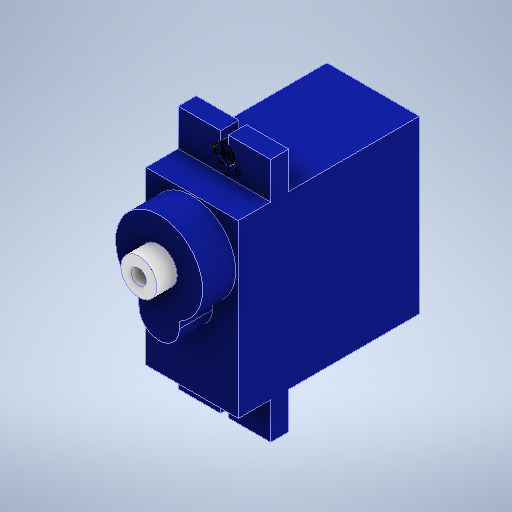
# Autodesk Inventor part: SG90 Servo
Saved by Autodesk Inventor 2025.1 (Build 291241000, 241)
## iProperties
Created: 2024-10-27
Part Number: SG90 Servo
Material: Generic
Document SubType Name: Modeling
Designer: jerem
Density: 1 g/cm^3
Appearance: Default
Author: jerem
Autodesk Inventor part; units mm, degrees
ref_plane "YZ Plane" through (0, 0, 0) normal (1, 0, 0) x (0, 1, 0)
ref_plane "XZ Plane" through (0, 0, 0) normal (0, 1, 0) x (-1, 0, 0)
ref_plane "XY Plane" through (0, 0, 0) normal (0, 0, 1) x (1, 0, 0)
sketch "Sketch1" plane through (0, 0, 0) normal (0, 0, 1) x (1, 0, 0)
  line L0 (6.15, -11.4) -> (-6.15, -11.4)
  line L1 (-6.15, -11.4) -> (-6.15, 11.4)
  line L2 (-6.15, 11.4) -> (6.15, 11.4)
  line L3 (6.15, 11.4) -> (6.15, -11.4)
  line L4 (6.15, -11.4) -> (-6.15, 11.4) construction
  line L5 (-6.15, -11.4) -> (6.15, 11.4) construction
  line L6 (-6.15, 11.4) -> (-6.15, 16.3)
  line L7 (6.15, 16.3) -> (6.15, 11.4)
  line L8 (-6.15, -11.4) -> (-6.15, -16.3)
  line L9 (6.15, -16.3) -> (6.15, -11.4)
  arc A0 (-0.5, 15.1) -> (0.5, 15.1) centre (0, 13.9) ccw
  line L10 (0, 13.9) -> (0, 11.4) construction
  line L11 (-0.5, 16.3) -> (-0.5, 15.1)
  line L12 (0.5, 15.1) -> (0.5, 16.3)
  line L13 (-0.5, 15.1) -> (0.5, 15.1) construction
  line L14 (0, 13.9) -> (0, 15.1) construction
  line L15 (-6.15, 16.3) -> (-0.5, 16.3)
  line L16 (0.5, 16.3) -> (6.15, 16.3)
  arc A1 (0.5, -15.1) -> (-0.5, -15.1) centre (0, -13.9) ccw
  line L17 (-0.5, -15.1) -> (-0.5, -16.3)
  line L18 (0.5, -15.1) -> (0.5, -16.3)
  line L19 (-0.5, -15.1) -> (0.5, -15.1) construction
  line L20 (0, -15.1) -> (0, -13.9) construction
  line L21 (0, -13.9) -> (0, -11.4) construction
  line L22 (-6.15, -16.3) -> (-0.5, -16.3)
  line L23 (0.5, -16.3) -> (6.15, -16.3)
  line L24 (0, 11.4) -> (0, 5.4) construction
  circle A2 centre (0, 5.4) radius 1
  circle A3 centre (0, 5.4) radius 2.4
  arc A4 (-2.7, -0.6) -> (2.7, -0.6) centre (0, -0.6) ccw
  line L25 (0, 5.4) -> (0, -0.6) construction
  line L26 (-2.7, -0.6) -> (-2.7, 0.2668)
  line L27 (2.7, -0.6) -> (2.7, 0.2668)
  arc A5 (2.7, 0.2668) -> (-2.7, 0.2668) centre (0, 5.4) ccw
  point P0 (0, 0)
  dimension "d0" = 22.8
  dimension "d1" = 12.3
  dimension "d4" = 2.6
  dimension "d5" = 2.5
  dimension "d6" = 1
  dimension "d7" = 4.9
  dimension "d8" = 2.5
  dimension "d9" = 1
  dimension "d10" = 2.6
  dimension "d11" = 4.9
  dimension "d14" = 6
  dimension "d15" = 2
  dimension "d16" = 4.8
  dimension "d17" = 5.4
  dimension "d18" = 6
  dimension "d19" = 5.8
  constraints: 57 end point, 15 perpendicular, 10 vertical, 8 point on circle, 6 centre point, 6 midpoint, 3 horizontal, 3 parallel, 2 coincident, 2 collinear, 2 tangent
  measures "d0" distance of L0.end L1.end
  measures "d1" distance of L1.end L2.end
  measures "d4" diameter of A0
  measures "d5" distance of L10.start L10.end
  measures "d6" distance between parallel lines of L12 L11
  measures "d7" distance between parallel lines of L2 L16
  measures "d8" distance of L20.end L21.end
  measures "d9" distance between parallel lines of L18 L17
  measures "d10" diameter of A1
  measures "d11" distance between parallel lines of L0 L23
  measures "d14" distance of L10.end L24.end
  measures "d15" diameter of A2
  measures "d16" diameter of A3
  measures "d17" diameter of A4
  measures "d18" distance of L25.start L25.end
  measures "d19" radius of A5
extrude "Extrusion1" add sketch "Sketch1" against normal blind 17.4 contours L0 L1 L2 L3 | A2 | A3 | L26 A5 L27 A4
extrude "Extrusion2" add sketch "Sketch1" along normal blind 2.4 contours L9 L23 L18 A1 L17 L22 L8 L0 | L0 L1 L2 L3 | L2 L6 L15 L11 A0 L12 L16 L7 | A2 | A3 | L26 A5 L27 A4
extrude "Extrusion3" add sketch "Sketch1" along normal blind 4.3 from surface at 2.4 contours L0 L1 L2 L3 | A2 | A3 | L26 A5 L27 A4
extrude "Extrusion4" add sketch "Sketch1" along normal blind 4.4 from surface at 6.7 contours A2 | A3 | L26 A5 L27 A4
extrude "Extrusion5" add sketch "Sketch1" along normal blind 2.7 from surface at 11.1 contours A3
sketch "Sketch2" plane through (0, 5.4, 11.1) normal (0, 0, 1) x (1, 0, 0)
  arc A0 (2.7, -5.1332) -> (-2.7, -5.1332) centre (0, 0) ccw projected
  line L0 (2.7, -5.1332) -> (2.7, -6) projected
  line L1 (-2.7, -6) -> (-2.7, -5.1332) projected
  arc A1 (-2.7, -6) -> (2.7, -6) centre (0, -6) ccw projected
  line L2 (6.15, -16.8) -> (-6.15, -16.8) projected
  line L3 (-6.15, -16.8) -> (6.15, -16.8) projected
  line L4 (6.15, -16.8) -> (-6.15, -16.8) projected
  line L5 (6.15, 6) -> (6.15, -16.8) projected
  line L6 (-6.15, 6) -> (6.15, 6) projected
  line L7 (-6.15, -16.8) -> (-6.15, 6) projected
  arc A2 (-2.7, -6) -> (2.7, -6) centre (0, -6) ccw projected
  line L8 (-2.7, -6) -> (-2.7, -5.1332) projected
  arc A3 (2.7, -5.1332) -> (-2.7, -5.1332) centre (0, 0) ccw projected
  line L9 (2.7, -5.1332) -> (2.7, -6) projected
  line L10 (-6.15, -16.8) -> (-6.15, 6) projected
  line L11 (6.15, -16.8) -> (-6.15, -16.8) projected
  line L12 (6.15, 6) -> (6.15, -16.8) projected
  line L13 (-6.15, 6) -> (6.15, 6) projected
  line L14 (-6.15, -16.8) -> (-6.15, 6) projected
  line L15 (-6.15, -16.8) -> (-6.15, -21.7) projected
  line L16 (-6.15, -16.8) -> (-6.15, -21.7) projected
  line L17 (-6.15, -16.8) -> (-6.15, 6) projected
  line L18 (-6.15, 10.9) -> (-6.15, 6) projected
  line L19 (-6.15, 10.9) -> (-6.15, 6) projected
  line L20 (6.15, 6) -> (6.15, -16.8) projected
  line L21 (6.15, -21.7) -> (6.15, -16.8) projected
  line L22 (6.15, -21.7) -> (6.15, -16.8) projected
  line L23 (6.15, 6) -> (6.15, -16.8) projected
  line L24 (6.15, 6) -> (6.15, 10.9) projected
  line L25 (6.15, 6) -> (6.15, 10.9) projected
  line L26 (6.15, -16.8) -> (-6.15, -16.8) projected
  line L27 (-6.15, -16.8) -> (-6.15, 6) projected
  line L28 (-6.15, 6) -> (6.15, 6) projected
  line L29 (6.15, 6) -> (6.15, -16.8) projected
  line L30 (-6.15, -16.8) -> (-6.15, 6) projected
  line L31 (6.15, 6) -> (6.15, -16.8) projected
  line L32 (-6.15, 6) -> (6.15, 6) projected
  line L33 (-6.15, -16.8) -> (6.15, -16.8) projected
  line L34 (6.15, -16.8) -> (-6.15, -16.8) projected
  line L35 (6.15, -16.8) -> (-6.15, -16.8) projected
  line L36 (6.15, -16.8) -> (-6.15, -16.8) projected
  line L37 (6.15, -21.7) -> (6.15, -16.8) projected
  line L38 (6.15, -21.7) -> (6.15, -16.8) projected
  line L39 (0.5, -20.5) -> (0.5, -21.7) projected
  line L40 (0.5, -20.5) -> (0.5, -21.7) projected
  line L41 (0.5, -20.5) -> (0.5, -21.7) projected
  line L42 (0.5, -21.7) -> (6.15, -21.7) projected
  line L43 (0.5, -21.7) -> (6.15, -21.7) projected
  line L44 (-6.15, -16.8) -> (-6.15, -21.7) projected
  line L45 (6.15, -16.8) -> (-6.15, -16.8) projected
  line L46 (-6.15, -16.8) -> (-6.15, -21.7) projected
  line L47 (-6.15, -21.7) -> (-0.5, -21.7) projected
  line L48 (-0.5, -21.7) -> (-0.5, -20.5) projected
  arc A4 (0.5, -20.5) -> (-0.5, -20.5) centre (0, -19.3) ccw projected
  line L49 (0.5, -20.5) -> (0.5, -21.7) projected
  line L50 (0.5, -21.7) -> (6.15, -21.7) projected
  line L51 (6.15, -21.7) -> (6.15, -16.8) projected
  line L52 (-6.15, -16.8) -> (6.15, -16.8) projected
  line L53 (6.15, -21.7) -> (6.15, -16.8) projected
  line L54 (0.5, -21.7) -> (6.15, -21.7) projected
  line L55 (0.5, -20.5) -> (0.5, -21.7) projected
  arc A5 (0.5, -20.5) -> (-0.5, -20.5) centre (0, -19.3) ccw projected
  line L56 (-0.5, -21.7) -> (-0.5, -20.5) projected
  line L57 (-6.15, -21.7) -> (-0.5, -21.7) projected
  line L58 (-6.15, -16.8) -> (-6.15, -21.7) projected
  line L59 (-6.15, -16.8) -> (-6.15, -21.7) projected
  line L60 (6.15, -16.8) -> (-6.15, -16.8) projected
  line L61 (-6.15, -21.7) -> (-0.5, -21.7) projected
  line L62 (-6.15, -21.7) -> (-0.5, -21.7) projected
  line L63 (-6.15, -21.7) -> (-0.5, -21.7) projected
  line L64 (0.5, -21.7) -> (6.15, -21.7) projected
  line L65 (-6.15, -21.7) -> (-0.5, -21.7) projected
  line L66 (-0.5, -21.7) -> (-0.5, -20.5) projected
  line L67 (-0.5, -21.7) -> (-0.5, -20.5) projected
  line L68 (-0.5, -21.7) -> (-0.5, -20.5) projected
  line L69 (-0.5, -21.7) -> (-0.5, -20.5) projected
  line L70 (0.5, -21.7) -> (6.15, -21.7) projected
  line L71 (-6.15, 10.9) -> (-6.15, 6) projected
  line L72 (-6.15, 10.9) -> (-6.15, 6) projected
  line L73 (6.15, 6) -> (6.15, 10.9) projected
  line L74 (6.15, 10.9) -> (0.5, 10.9) projected
  line L75 (0.5, 10.9) -> (0.5, 9.7) projected
  arc A6 (-0.5, 9.7) -> (0.5, 9.7) centre (0, 8.5) ccw projected
  line L76 (-0.5, 9.7) -> (-0.5, 10.9) projected
  line L77 (-0.5, 10.9) -> (-6.15, 10.9) projected
  line L78 (-6.15, 6) -> (6.15, 6) projected
  line L79 (-6.15, 6) -> (6.15, 6) projected
  line L80 (-6.15, 6) -> (6.15, 6) projected
  line L81 (6.15, 6) -> (6.15, 10.9) projected
  line L82 (6.15, 10.9) -> (0.5, 10.9) projected
  line L83 (0.5, 10.9) -> (0.5, 9.7) projected
  arc A7 (-0.5, 9.7) -> (0.5, 9.7) centre (0, 8.5) ccw projected
  arc A8 (0.5, -20.5) -> (-0.5, -20.5) centre (0, -19.3) ccw projected
  arc A9 (0.5, -20.5) -> (-0.5, -20.5) centre (0, -19.3) ccw projected
  arc A10 (0.5, -20.5) -> (-0.5, -20.5) centre (0, -19.3) ccw projected
  arc A11 (0.5, -20.5) -> (-0.5, -20.5) centre (0, -19.3) ccw projected
  circle A12 centre (0, 0) radius 2.4 projected
  circle A13 centre (0, 0) radius 2.4 projected
  circle A14 centre (0, 0) radius 1 projected
  circle A15 centre (0, 0) radius 1 projected
  arc A16 (-2.7, -6) -> (2.7, -6) centre (0, -6) ccw projected
  line L84 (2.7, -5.1332) -> (2.7, -6) projected
  arc A17 (2.7, -5.1332) -> (-2.7, -5.1332) centre (0, 0) ccw projected
  line L85 (-2.7, -6) -> (-2.7, -5.1332) projected
  arc A18 (2.7, -5.1332) -> (-2.7, -5.1332) centre (0, 0) ccw projected
  arc A19 (2.7, -5.1332) -> (-2.7, -5.1332) centre (0, 0) ccw projected
  arc A20 (-2.7, -6) -> (2.7, -6) centre (0, -6) ccw projected
  line L86 (2.7, -5.1332) -> (2.7, -6) projected
  arc A21 (2.7, -5.1332) -> (-2.7, -5.1332) centre (0, 0) ccw projected
  line L87 (-2.7, -6) -> (-2.7, -5.1332) projected
  circle A22 centre (0, 0) radius 2.4 projected
  arc A23 (-2.7, -6) -> (2.7, -6) centre (0, -6) ccw projected
  arc A24 (-2.7, -6) -> (2.7, -6) centre (0, -6) ccw projected
  line L88 (-2.7, -6) -> (-2.7, -5.1332) projected
  line L89 (-2.7, -6) -> (-2.7, -5.1332) projected
  line L90 (2.7, -5.1332) -> (2.7, -6) projected
  line L91 (2.7, -5.1332) -> (2.7, -6) projected
  circle A25 centre (0, 0) radius 1 projected
  circle A26 centre (0, 0) radius 1 projected
  circle A27 centre (0, 0) radius 1 projected
  circle A28 centre (0, 0) radius 1 projected
  circle A29 centre (0, 0) radius 2.4 projected
  circle A30 centre (0, 0) radius 2.4 projected
  circle A31 centre (0, 0) radius 2.4 projected
  line L92 (0.5, -20.5) -> (0.5, -21.7) projected
  line L93 (6.15, 6) -> (-6.15, 6) projected
  line L94 (6.15, 6) -> (-6.15, 6) projected
  line L95 (-6.15, 10.9) -> (-6.15, 6) projected
  line L96 (-0.5, 10.9) -> (-6.15, 10.9) projected
  line L97 (-0.5, 9.7) -> (-0.5, 10.9) projected
  arc A32 (-0.5, 9.7) -> (0.5, 9.7) centre (0, 8.5) ccw projected
  line L98 (0.5, 10.9) -> (0.5, 9.7) projected
  line L99 (6.15, 10.9) -> (0.5, 10.9) projected
  line L100 (6.15, 6) -> (6.15, 10.9) projected
  line L101 (-6.15, 6) -> (6.15, 6) projected
  line L102 (6.15, 6) -> (6.15, 10.9) projected
  line L103 (6.15, 10.9) -> (0.5, 10.9) projected
  line L104 (0.5, 10.9) -> (0.5, 9.7) projected
  arc A33 (-0.5, 9.7) -> (0.5, 9.7) centre (0, 8.5) ccw projected
  line L105 (-0.5, 9.7) -> (-0.5, 10.9) projected
  line L106 (-0.5, 10.9) -> (-6.15, 10.9) projected
  line L107 (-6.15, 10.9) -> (-6.15, 6) projected
  line L108 (6.15, 6) -> (-6.15, 6) projected
  line L109 (-6.15, 6) -> (6.15, 6) projected
  line L110 (6.15, 10.9) -> (0.5, 10.9) projected
  line L111 (6.15, 10.9) -> (0.5, 10.9) projected
  arc A34 (-0.5, 9.7) -> (0.5, 9.7) centre (0, 8.5) ccw projected
  arc A35 (-0.5, 9.7) -> (0.5, 9.7) centre (0, 8.5) ccw projected
  line L112 (0.5, 10.9) -> (0.5, 9.7) projected
  line L113 (0.5, 10.9) -> (0.5, 9.7) projected
  line L114 (-0.5, 9.7) -> (-0.5, 10.9) projected
  line L115 (-0.5, 9.7) -> (-0.5, 10.9) projected
  line L116 (-0.5, 9.7) -> (-0.5, 10.9) projected
  line L117 (-0.5, 10.9) -> (-6.15, 10.9) projected
  line L118 (-0.5, 10.9) -> (-6.15, 10.9) projected
  line L119 (-0.5, 10.9) -> (-6.15, 10.9) projected
  point P0 (0, -5.4)
  dimension "d30" = 4.8
  dimension "d31" = 8.5
  dimension "d32" = 19.3
  dimension "d33" = 1.3
  dimension "d34" = 6
  dimension "d35" = 16.8
  constraints: 23 other
  measures "d30" diameter of A12
  measures "d31" distance of A6.centre A0.centre
  measures "d32" distance of A4.centre A0.centre
  measures "d33" radius of A6
  measures "d34" distance from line of L6 A0.centre
  measures "d35" distance from line of L2 A0.centre
sketch "Sketch3" plane through (0, 0, 2.4) normal (0, 0, 1) x (1, 0, 0)
  circle A0 centre (0, 13.9) radius 1.3
  arc A1 (-0.5, 15.1) -> (0.5, 15.1) centre (0, 13.9) ccw projected
  point P0 (0, 0)
  dimension "d36" = 0
  dimension "d37" = 2.6
  constraints: 1 centre point
  measures "d36" distance of A0.centre A1.centre
  measures "d37" diameter of A0
sketch "Sketch4" plane through (0, 0, 2.4) normal (0, 0, 1) x (1, 0, 0)
  arc A0 (0.5, -15.1) -> (-0.5, -15.1) centre (0, -13.9) ccw projected
  circle A1 centre (0, -13.9) radius 1.3
  point P0 (0, 0)
  constraints: 1 centre point, 1 coincident
equation "\"d8\" = d5"
equation "\"d9\" = d6"
equation "\"d10\" = d4"
equation "\"d11\" = d7"
equation "\"d3\" = d2"
equation "\"d2\" = 4.9"
body "Solid1"
